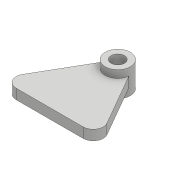
# Autodesk Inventor part: Offset
Saved by Autodesk Inventor 2022 Beta2 (Build 260130000, 130) ContinuousBuild 0
## iProperties
Created: 2016-01-25
Part Number: Offset
Material: Generic
Document SubType Name: Modeling
Designer: jmacmillan
Density: 1 g/cm^3
Appearance: Default
Author: jmacmillan
Autodesk Inventor part; units mm, degrees
ref_plane "YZ Plane" through (0, 0, 0) normal (1, 0, 0) x (0, 1, 0)
ref_plane "XZ Plane" through (0, 0, 0) normal (0, 1, 0) x (-1, 0, 0)
ref_plane "XY Plane" through (0, 0, 0) normal (0, 0, 1) x (1, 0, 0)
sketch "Sketch1" plane through (0, 0, 0) normal (0, 0, 1) x (1, 0, 0)
  arc A0 (5.1962, 37.641) -> (-5.1962, 37.641) centre (0, 34.641) ccw
  arc A1 (-25.1962, 3) -> (-20, -6) centre (-20, 0) ccw
  arc A2 (20, -6) -> (25.1962, 3) centre (20, 0) ccw
  line L0 (-5.1962, 37.641) -> (-25.1962, 3)
  line L1 (-20, -6) -> (20, -6)
  line L2 (25.1962, 3) -> (5.1962, 37.641)
  circle A3 centre (0, 34.641) radius 7.5
  line L3 (0, 52.0692) -> (0, -17.4282) projected
  line L4 (-38.9119, 0) -> (38.9119, 0) projected
  circle A4 centre (0, 34.641) radius 4
  point P0 (0, 0)
  dimension "d0" = 6
  dimension "d1" = 40
  dimension "d2" = 15
  dimension "d7" = 8
  constraints: 8 point on circle, 6 end point, 6 tangent, 5 centre point, 5 point on line, 2 coincident, 2 equal length, 2 equal radius
  measures "d0" radius of A2
  measures "d1" distance of L0.start L0.end
  measures "d2" diameter of A3
  measures "d7" diameter of A4
extrude "Extrusion1" add sketch "Sketch1" along normal mid plane 6 contours L2 A3 L3 A4 A0 | L3 A4 A3 L0 A0 | L2 A2 L4 L3 A3 | A4 L3 | L3 A4 | L3 L4 A1 L0 A3 | A2 L1 L3 L4 | L3 L1 A1 L4
extrude "Extrusion2" add sketch "Sketch1" along normal mid plane 15 contours L2 A3 L3 A4 A0 | A0 L3 A3 L2 | L3 A4 A3 L0 A0 | A0 L0 A3 L3 | A4 L3 | L3 A4
extrude "Extrusion3" cut sketch "Sketch1" along normal through all both and the other way through all contours A4 L3 | L3 A4
body "Solid1"
